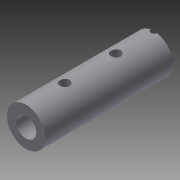
# Autodesk Inventor part: shaft_to_dc_coupler
Saved by Autodesk Inventor 2015 (Build 190159000, 159)
## iProperties
Created: 2017-09-26
Part Number: shaft_to_dc_coupler
Material: Generic
Document SubType Name: Modeling
Designer: Anshul
Density: 1 g/cm^3
Appearance: Default
Author: Anshul
Autodesk Inventor part; units mm, degrees
ref_plane "YZ Plane" through (0, 0, 0) normal (1, 0, 0) x (0, 1, 0)
ref_plane "XZ Plane" through (0, 0, 0) normal (0, 1, 0) x (-1, 0, 0)
ref_plane "XY Plane" through (0, 0, 0) normal (0, 0, 1) x (1, 0, 0)
sketch "Sketch1" plane through (0, 0, 0) normal (0, 1, 0) x (-1, 0, 0)
  line L0 (0, 0) -> (3, 0)
  line L1 (3, 0) -> (3, -20)
  line L2 (3, -20) -> (0, -20)
  line L3 (0, -20) -> (0, 0)
  line L4 (0, 0) -> (0, -8)
  circle A0 centre (0, -8) radius 1.55
  line L5 (3, 0) -> (6, 0)
  line L6 (6, 0) -> (6, -20)
  line L7 (6, -20) -> (3, -20)
  line L8 (0, 0) -> (3.15, 0)
  line L9 (3.15, 0) -> (3.15, 20)
  line L10 (3.15, 20) -> (0, 20)
  line L11 (0, 20) -> (0, 0)
  line L12 (0, 0) -> (0, 8)
  circle A1 centre (0, 8) radius 1.55
  line L13 (3.15, 20) -> (6, 20)
  line L14 (6, 20) -> (6, 0)
  circle A2 centre (0, -20) radius 1
  dimension "d0" = 3
  dimension "d1" = 20
  dimension "d2" = 3
  dimension "d3" = 8
  dimension "d4" = 3.1
  dimension "d5" = 3
  dimension "d6" = 3.15
  dimension "d7" = 20
  dimension "d8" = 8
  dimension "d9" = 3.1
  dimension "d11" = 2
  constraints: 30 end point, 8 perpendicular, 3 centre point, 3 coincident, 3 horizontal, 3 point on line
  measures "d0" distance of L0.start L0.end
  measures "d1" distance of L0.end L1.end
  measures "d2" distance of L1.end L2.end
  measures "d3" distance of L0.start L4.end
  measures "d4" diameter of A0
  measures "d5" distance of L0.end L5.end
  measures "d6" distance of L0.start L8.end
  measures "d7" distance of L8.end L9.end
  measures "d8" distance of L0.start L12.end
  measures "d9" diameter of A1
  measures "d11" diameter of A2
revolve "Revolution1" add sketch "Sketch1" angle 360 about axis through (0, 0, 20) along (0, 0, -1) contours L5 L6 L7 L1 | L9 L13 L14 L5
extrude "Extrusion1" cut sketch "Sketch1" along normal mid plane 20 contours A0 L3 | L3 A0 | A1 L11 | L11 A1 | A2 L3 L2 | L2 L3 A2
body "Solid1"
